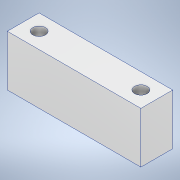
# Autodesk Inventor part: Espaciador Sub Inferior
Saved by Autodesk Inventor 2020 (Build 240168000, 168)
## iProperties
Created: 2020-05-16
Part Number: Espaciador Sub Inferior
Material: Aluminum 6061
Document SubType Name: Modeling
Designer: Dante
Density: 2.7 g/cm^3
Appearance: Aluminum - Flat
Mass: 15.9921 g
Surface Area: 27.2673 cm^2
Volume: 5.92301 cm^3
Author: Dante
Autodesk Inventor part; units mm, degrees
ref_plane "YZ Plane" through (0, 0, 0) normal (1, 0, 0) x (0, 1, 0)
ref_plane "XZ Plane" through (0, 0, 0) normal (0, 1, 0) x (-1, 0, 0)
ref_plane "XY Plane" through (0, 0, 0) normal (0, 0, 1) x (1, 0, 0)
sketch "Sketch1" plane through (0, 0, 0) normal (0, 0, 1) x (1, 0, 0)
  line L0 (50, -5) -> (50, 11)
  line L1 (50, 11) -> (8, 11)
  line L2 (8, -5) -> (8, 11)
  line L3 (8, -5) -> (50, -5)
  dimension "d1" = 16
  dimension "d47" = 42
  constraints: 8 end point, 1 horizontal, 1 perpendicular, 1 vertical
  measures "d1" distance of L0.start L0.end
  measures "d47" distance of L2.start L0.start
extrude "Extrusion3" add sketch "Sketch1" along normal blind 10
sketch "Sketch6" plane through (8, 11, 0) normal (0, 1, 0) x (1, 0, 0)
  circle A0 centre (5, -5) radius 2
  circle A1 centre (37, -5) radius 2
  line L0 (42, 0) -> (0, 0) projected
  line L1 (42, 0) -> (42, -10) projected
  line L2 (0, 0) -> (0, -10) projected
  dimension "d48" = 4
  dimension "d49" = 4
  dimension "d50" = 5
  dimension "d51" = 5
  dimension "d52" = 5
  dimension "d53" = 5
  constraints: 2 centre point
  measures "d48" diameter of A0
  measures "d49" diameter of A1
  measures "d50" distance from line of L0 A1.centre
  measures "d51" distance from line of A1.centre L1
  measures "d52" distance from line of L0 A0.centre
  measures "d53" distance from line of L2 A0.centre
extrude "Extrusion7" cut sketch "Sketch6" against normal blind 50
body "Solid1"
